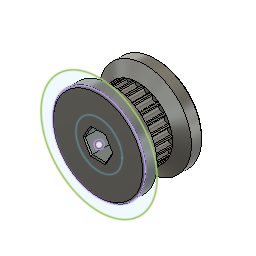
HTD Flanged Pulley (Autodesk Fusion 360 design; units mm, degrees)
Autodesk Fusion 360 part; units mm, degrees
sketch "Basic Outline" plane through (0, 0, 0) normal (0, 0, 1) x (1, 0, 0) in component "HTD 5M Pulley"
  circle A0 centre (0, 0) radius 18.5271
  line L0 (0, 0) -> (0, 17.9921) construction
  arc A1 (-1.525, 17.9914) -> (-2.0015, 18.4187) centre (-1.955, 17.9912) ccw
  arc A2 (-1.525, 17.9914) -> (1.525, 17.9914) centre (0, 17.9921) ccw
  arc A3 (2.0015, 18.4187) -> (1.525, 17.9914) centre (1.955, 17.9912) ccw
  dimension "d12" = 3.05
  dimension "d19" = 37.0542
  dimension "d20" = 16.4671
  dimension "d21" = 0.43
  constraint coincident A0.centre L0.start
  constraint coincident L0.end A2.centre
  constraint tangent A1 A2
  constraint tangent A0 A1
  constraint coincident A0 A1.end
  constraint vertical L0
  constraint tangent A0 A3
  constraint tangent A2 A3
  constraint coincident A0 A3.start
  constraint equal A1 A3
  measures "d12" diameter of A2
  measures "d19" diameter of A0
  measures "d20" distance of A0.centre A2
  measures "d21" radius of A1
extrude "Extrude1" add sketch "Basic Outline" along normal blind 5.5 in component "HTD 5M Pulley"
extrude "Extrude2" cut sketch "Basic Outline" along normal blind 5.5 contours A0 A1 A2 A3 picked at (-0.038, 17.8338) in component "HTD 5M Pulley"
pattern_circular "C-Pattern1" count 24 over 360 about axis through (0, 0, 1.75) along (0, 0, 1) of "Extrude2" in component "HTD 5M Pulley"
sketch "Flange" plane through (0, 0, 5.5) normal (0, 0, 1) x (1, 0, 0) in component "HTD 5M Pulley"
  arc A0 (2.0015, 18.4187) -> (1.525, 17.9914) centre (1.955, 17.9912) ccw
  arc A1 (-1.525, 17.9914) -> (1.525, 17.9914) centre (0, 17.9921) ccw
  arc A2 (-1.525, 17.9914) -> (-2.0015, 18.4187) centre (-1.955, 17.9912) ccw
  arc A3 (-2.0015, 18.4187) -> (-2.8338, 18.3091) centre (0, 0) ccw
  arc A4 (-2.8338, 18.3091) -> (-3.1835, 17.773) centre (-2.7681, 17.8841) ccw
  arc A5 (-6.1295, 16.9836) -> (-3.1835, 17.773) centre (-4.6567, 17.379) ccw
  arc A6 (-6.1295, 16.9836) -> (-6.7004, 17.2731) centre (-6.5448, 16.8722) ccw
  arc A7 (-6.7004, 17.2731) -> (-7.476, 16.9518) centre (0, 0) ccw
  arc A8 (-7.476, 16.9518) -> (-7.675, 16.3435) centre (-7.3025, 16.5583) ccw
  arc A9 (-10.3164, 14.8185) -> (-7.675, 16.3435) centre (-8.996, 15.5816) ccw
  arc A10 (-10.3164, 14.8185) -> (-10.9426, 14.9503) centre (-10.6887, 14.6033) ccw
  arc A11 (-10.9426, 14.9503) -> (-11.6087, 14.4392) centre (0, 0) ccw
  arc A12 (-11.6087, 14.4392) -> (-11.6435, 13.8002) centre (-11.3393, 14.1041) ccw
  arc A13 (-13.8002, 11.6435) -> (-11.6435, 13.8002) centre (-12.7223, 12.7223) ccw
  arc A14 (-13.8002, 11.6435) -> (-14.4392, 11.6087) centre (-14.1041, 11.3393) ccw
  arc A15 (-14.4392, 11.6087) -> (-14.9503, 10.9426) centre (0, 0) ccw
  arc A16 (-14.9503, 10.9426) -> (-14.8185, 10.3164) centre (-14.6033, 10.6887) ccw
  arc A17 (-16.3435, 7.675) -> (-14.8185, 10.3164) centre (-15.5816, 8.996) ccw
  arc A18 (-16.3435, 7.675) -> (-16.9518, 7.476) centre (-16.5583, 7.3025) ccw
  arc A19 (-16.9518, 7.476) -> (-17.2731, 6.7004) centre (0, 0) ccw
  arc A20 (-17.2731, 6.7004) -> (-16.9836, 6.1295) centre (-16.8722, 6.5448) ccw
  arc A21 (-17.773, 3.1835) -> (-16.9836, 6.1295) centre (-17.379, 4.6567) ccw
  arc A22 (-17.773, 3.1835) -> (-18.3091, 2.8338) centre (-17.8841, 2.7681) ccw
  arc A23 (-18.3091, 2.8338) -> (-18.4187, 2.0015) centre (0, 0) ccw
  arc A24 (-18.4187, 2.0015) -> (-17.9914, 1.525) centre (-17.9912, 1.955) ccw
  arc A25 (-17.9914, -1.525) -> (-17.9914, 1.525) centre (-17.9921, 0) ccw
  arc A26 (-17.9914, -1.525) -> (-18.4187, -2.0015) centre (-17.9912, -1.955) ccw
  arc A27 (-18.4187, -2.0015) -> (-18.3091, -2.8338) centre (0, 0) ccw
  arc A28 (-18.3091, -2.8338) -> (-17.773, -3.1835) centre (-17.8841, -2.7681) ccw
  arc A29 (-16.9836, -6.1295) -> (-17.773, -3.1835) centre (-17.379, -4.6567) ccw
  arc A30 (-16.9836, -6.1295) -> (-17.2731, -6.7004) centre (-16.8722, -6.5448) ccw
  arc A31 (-17.2731, -6.7004) -> (-16.9518, -7.476) centre (0, 0) ccw
  arc A32 (-16.9518, -7.476) -> (-16.3435, -7.675) centre (-16.5583, -7.3025) ccw
  arc A33 (-14.8185, -10.3164) -> (-16.3435, -7.675) centre (-15.5816, -8.996) ccw
  arc A34 (-14.8185, -10.3164) -> (-14.9503, -10.9426) centre (-14.6033, -10.6887) ccw
  arc A35 (-14.9503, -10.9426) -> (-14.4392, -11.6087) centre (0, 0) ccw
  arc A36 (-14.4392, -11.6087) -> (-13.8002, -11.6435) centre (-14.1041, -11.3393) ccw
  arc A37 (-11.6435, -13.8002) -> (-13.8002, -11.6435) centre (-12.7223, -12.7223) ccw
  arc A38 (-11.6435, -13.8002) -> (-11.6087, -14.4392) centre (-11.3393, -14.1041) ccw
  arc A39 (-11.6087, -14.4392) -> (-10.9426, -14.9503) centre (0, 0) ccw
  arc A40 (-10.9426, -14.9503) -> (-10.3164, -14.8185) centre (-10.6887, -14.6033) ccw
  arc A41 (-7.675, -16.3435) -> (-10.3164, -14.8185) centre (-8.996, -15.5816) ccw
  arc A42 (-7.675, -16.3435) -> (-7.476, -16.9518) centre (-7.3025, -16.5583) ccw
  arc A43 (-7.476, -16.9518) -> (-6.7004, -17.2731) centre (0, 0) ccw
  arc A44 (-6.7004, -17.2731) -> (-6.1295, -16.9836) centre (-6.5448, -16.8722) ccw
  arc A45 (-3.1835, -17.773) -> (-6.1295, -16.9836) centre (-4.6567, -17.379) ccw
  arc A46 (-3.1835, -17.773) -> (-2.8338, -18.3091) centre (-2.7681, -17.8841) ccw
  arc A47 (-2.8338, -18.3091) -> (-2.0015, -18.4187) centre (0, 0) ccw
  arc A48 (-2.0015, -18.4187) -> (-1.525, -17.9914) centre (-1.955, -17.9912) ccw
  arc A49 (1.525, -17.9914) -> (-1.525, -17.9914) centre (0, -17.9921) ccw
  arc A50 (1.525, -17.9914) -> (2.0015, -18.4187) centre (1.955, -17.9912) ccw
  arc A51 (2.0015, -18.4187) -> (2.8338, -18.3091) centre (0, 0) ccw
  arc A52 (2.8338, -18.3091) -> (3.1835, -17.773) centre (2.7681, -17.8841) ccw
  arc A53 (6.1295, -16.9836) -> (3.1835, -17.773) centre (4.6567, -17.379) ccw
  arc A54 (6.1295, -16.9836) -> (6.7004, -17.2731) centre (6.5448, -16.8722) ccw
  arc A55 (6.7004, -17.2731) -> (7.476, -16.9518) centre (0, 0) ccw
  arc A56 (7.476, -16.9518) -> (7.675, -16.3435) centre (7.3025, -16.5583) ccw
  arc A57 (10.3164, -14.8185) -> (7.675, -16.3435) centre (8.996, -15.5816) ccw
  arc A58 (10.3164, -14.8185) -> (10.9426, -14.9503) centre (10.6887, -14.6033) ccw
  arc A59 (10.9426, -14.9503) -> (11.6087, -14.4392) centre (0, 0) ccw
  arc A60 (11.6087, -14.4392) -> (11.6435, -13.8002) centre (11.3393, -14.1041) ccw
  arc A61 (13.8002, -11.6435) -> (11.6435, -13.8002) centre (12.7223, -12.7223) ccw
  arc A62 (13.8002, -11.6435) -> (14.4392, -11.6087) centre (14.1041, -11.3393) ccw
  arc A63 (14.4392, -11.6087) -> (14.9503, -10.9426) centre (0, 0) ccw
  arc A64 (14.9503, -10.9426) -> (14.8185, -10.3164) centre (14.6033, -10.6887) ccw
  arc A65 (16.3435, -7.675) -> (14.8185, -10.3164) centre (15.5816, -8.996) ccw
  arc A66 (16.3435, -7.675) -> (16.9518, -7.476) centre (16.5583, -7.3025) ccw
  arc A67 (16.9518, -7.476) -> (17.2731, -6.7004) centre (0, 0) ccw
  arc A68 (17.2731, -6.7004) -> (16.9836, -6.1295) centre (16.8722, -6.5448) ccw
  arc A69 (17.773, -3.1835) -> (16.9836, -6.1295) centre (17.379, -4.6567) ccw
  arc A70 (17.773, -3.1835) -> (18.3091, -2.8338) centre (17.8841, -2.7681) ccw
  arc A71 (18.3091, -2.8338) -> (18.4187, -2.0015) centre (0, 0) ccw
  arc A72 (18.4187, -2.0015) -> (17.9914, -1.525) centre (17.9912, -1.955) ccw
  arc A73 (17.9914, 1.525) -> (17.9914, -1.525) centre (17.9921, 0) ccw
  arc A74 (17.9914, 1.525) -> (18.4187, 2.0015) centre (17.9912, 1.955) ccw
  arc A75 (18.4187, 2.0015) -> (18.3091, 2.8338) centre (0, 0) ccw
  arc A76 (18.3091, 2.8338) -> (17.773, 3.1835) centre (17.8841, 2.7681) ccw
  arc A77 (16.9836, 6.1295) -> (17.773, 3.1835) centre (17.379, 4.6567) ccw
  arc A78 (16.9836, 6.1295) -> (17.2731, 6.7004) centre (16.8722, 6.5448) ccw
  arc A79 (17.2731, 6.7004) -> (16.9518, 7.476) centre (0, 0) ccw
  arc A80 (16.9518, 7.476) -> (16.3435, 7.675) centre (16.5583, 7.3025) ccw
  arc A81 (14.8185, 10.3164) -> (16.3435, 7.675) centre (15.5816, 8.996) ccw
  arc A82 (14.8185, 10.3164) -> (14.9503, 10.9426) centre (14.6033, 10.6887) ccw
  arc A83 (14.9503, 10.9426) -> (14.4392, 11.6087) centre (0, 0) ccw
  arc A84 (14.4392, 11.6087) -> (13.8002, 11.6435) centre (14.1041, 11.3393) ccw
  arc A85 (11.6435, 13.8002) -> (13.8002, 11.6435) centre (12.7223, 12.7223) ccw
  arc A86 (11.6435, 13.8002) -> (11.6087, 14.4392) centre (11.3393, 14.1041) ccw
  arc A87 (11.6087, 14.4392) -> (10.9426, 14.9503) centre (0, 0) ccw
  arc A88 (10.9426, 14.9503) -> (10.3164, 14.8185) centre (10.6887, 14.6033) ccw
  arc A89 (7.675, 16.3435) -> (10.3164, 14.8185) centre (8.996, 15.5816) ccw
  arc A90 (7.675, 16.3435) -> (7.476, 16.9518) centre (7.3025, 16.5583) ccw
  arc A91 (7.476, 16.9518) -> (6.7004, 17.2731) centre (0, 0) ccw
  arc A92 (6.7004, 17.2731) -> (6.1295, 16.9836) centre (6.5448, 16.8722) ccw
  arc A93 (3.1835, 17.773) -> (6.1295, 16.9836) centre (4.6567, 17.379) ccw
  arc A94 (3.1835, 17.773) -> (2.8338, 18.3091) centre (2.7681, 17.8841) ccw
  arc A95 (2.8338, 18.3091) -> (2.0015, 18.4187) centre (0, 0) ccw
  circle A96 centre (0, 0) radius 18.5271 construction
  circle A97 centre (0, 0) radius 25.0271
  circle A98 centre (0, 0) radius 75.0271
  dimension "d58" = 6.5
  dimension "d59" = 50
  constraint concentric A96 A97
  measures "d58" distance of A96 A97
  measures "d59" distance of A97 A98
extrude "Extrude3" add sketch "Basic Outline" along normal blind 10.15 draft 60 from surface at 5.5 in component "HTD 5M Pulley"
extrude "Extrude4" cut sketch "Flange" along normal through all contours A98 in component "HTD 5M Pulley"
sketch "Hub" plane through (0, 0, 15.65) normal (0, 0, 1) x (1, 0, 0) in component "HTD 5M Pulley"
  circle A0 centre (0, 0) radius 12.5
  circle A1 centre (0, 0) radius 31.3722
  circle A2 centre (0, 0) radius 25.0271
  dimension "d64" = 25
  measures "d64" diameter of A0
extrude "Extrude7" add sketch "Hub" along normal blind 0.6 contours A0 in component "HTD 5M Pulley"
sketch "Axle and Bolts" plane through (0, 0, 16.25) normal (0, 0, 1) x (1, 0, 0) in component "HTD 5M Pulley"
  circle A0 centre (0, 0) radius 18.5271 construction
  line L0 (-3.7212, 6.4452) -> (-7.4423, 0)
  line L1 (-7.4423, 0) -> (-3.7212, -6.4453)
  line L2 (-3.7212, -6.4453) -> (3.7212, -6.4453)
  line L3 (3.7212, -6.4452) -> (7.4423, 0)
  line L4 (7.4423, 0) -> (3.7212, 6.4452)
  line L5 (3.7212, 6.4452) -> (-3.7212, 6.4452)
  circle A1 centre (0, 0) radius 21.0271
  line L6 (0, 0) -> (0, 11.9671) construction
  circle A2 centre (0, 0) radius 15
  circle A3 centre (0, 0) radius 12.5
  line L7 (3.7212, -6.4452) -> (7.5, -12.9904) construction
  line L8 (5.6106, -9.7178) -> (11.2212, 0)
  line L9 (11.2212, 0) -> (5.6106, 9.7178)
  line L10 (5.6106, 9.7178) -> (-5.6106, 9.7178)
  line L11 (-5.6106, 9.7178) -> (-11.2212, 0)
  line L12 (-11.2212, 0) -> (-5.6106, -9.7178)
  line L13 (-5.6106, -9.7178) -> (5.6106, -9.7178)
  line L14 (12.6068, 0) -> (6.3034, 10.9178)
  line L15 (6.3034, 10.9178) -> (-6.3034, 10.9178)
  line L16 (-6.3034, 10.9178) -> (-12.6068, 0)
  line L17 (-12.6068, 0) -> (-6.3034, -10.9178)
  line L18 (-6.3034, -10.9178) -> (6.3034, -10.9178)
  line L19 (6.3034, -10.9178) -> (12.6068, 0)
  point P0 (0, 11.9671)
  dimension "d60" = 6.4452
  dimension "d77" = 11.9671
  dimension "d83" = 1.2
  constraint coincident A0.centre A1.centre
  constraint coincident P0 L6.end
  constraint perpendicular L5 L6
  constraint vertical L6
  constraint coincident A2 L7.end
  constraint parallel L1 L7
  constraint coincident L7 L8.start
  constraint midpoint L7 L8.start
  measures "d60" distance of A0.centre L5
  measures "d77" distance of A0.centre L6.end
extrude "Extrude6" cut sketch "Axle and Bolts" against normal through all contours L0 L1 L2 L3 L4 L5 in component "HTD 5M Pulley"
chamfer "Chamfer1" distance 0.6 angle 45 6 edges at (5.5818, -3.2226, 16.25) (0, -6.4453, 16.25) (-5.5818, -3.2226, 16.25) (-5.5818, 3.2226, 16.25) (0, 6.4452, 16.25) (5.5818, 3.2226, 16.25) in component "HTD 5M Pulley"
mirror "Mirror1" about plane through (0, 0, 0) normal (0, 0, -1) of bodies 1 merged in component "HTD 5M Pulley"
extrude "Extrude9" add sketch "Hub" along normal up to surface (0.6 mm away) contours A2 in component "HTD 5M Pulley"
chamfer "Chamfer2" distance 0.9 angle 45 2 edges at (-23.3334, 9.0502, 16.25) (-23.3334, -9.0502, -15.65) in component "HTD 5M Pulley"
component "HTD 5M Pulley" placed x (1, 0, 0) y (0, 1, 0) z (0, 0, 1) at (0, 0, 0)
equation "NUM_TEETH = 24" comment "Number of teeth in the pulley"
equation "TOOTH_PITCH = 5 mm" comment "Belt pitch (ie: 5mm=HTD5)"
equation "zOutsideDia = 2 * ( ( NUM_TEETH * TOOTH_PITCH ) / ( PI * 2 ) - zPitchLineOffset )"
equation "zPitchLineOffset = 0.5715 mm"
equation "zToothDia = 2.06 mm"
equation "zMinorDia = zOutsideDia - 2 * zToothDia"
equation "zToothWidth = 3.05 mm"
equation "zToothRootDia = 0.86 mm"
equation "d12 = zToothWidth"
equation "d17 = TOOTH_WIDTH / 2"
equation "d19 = zOutsideDia"
equation "d20 = zMinorDia / 2"
equation "d21 = zToothRootDia / 2"
equation "d22 = d17"
equation "d24 = NUM_TEETH"
equation "TOOTH_WIDTH = 11 mm" comment "Width of the toothed part of the pulley"
equation "TOTAL_WIDTH = 14.5 mm + EXTRA_WIDTH" comment "Total width of the pulley at the hub"
equation "PRINTER_LAYER_HEIGHT = 0.3 mm" comment "Layer height of printer (typically 0.2mm or 0.3mm)"
equation "HUB_OFFSET = if(PRINTER_LAYER_HEIGHT >= 0.3 mm; PRINTER_LAYER_HEIGHT * 2; PRINTER_LAYER_HEIGHT * 3)" comment "Distant hub projects above rim (so rim won't scrape when pulley rotates)"
equation "FLANGE_ANGLE = 60 deg" comment "Typically 60 if printing with a hub offset, 80 otherwise"
equation "HEX_SHAFT_DIAMETER = 0.5075 in" comment "Hex shaft diameter + tolerance"
equation "d34 = ( TOTAL_WIDTH - TOOTH_WIDTH ) / 2 - HUB_OFFSET"
equation "d35 = FLANGE_ANGLE"
equation "FLANGE_MAX_HEIGHT = 2.5 mm + EXTRA_DIAMETER" comment "Max height of the flange"
equation "HUB_DIAMETER = 25 mm" comment "Diameter of the raised hub"
equation "NUM_BOLTS = 6" comment "Number of mounting bolts (edit feature to change type)"
equation "d54 = PRINTER_LAYER_HEIGHT * 2"
equation "d58 = FLANGE_MAX_HEIGHT"
equation "d60 = HEX_SHAFT_DIAMETER / 2"
equation "BOLT_RADIUS = min(( zOutsideDia + HUB_DIAMETER ) / 4; zMinorDia / 2 - 4.5 mm)" comment "Radius of the bolt circle (default is halfway between hub and rim)"
equation "d64 = HUB_DIAMETER"
equation "d65 = HUB_OFFSET"
equation "d77 = BOLT_RADIUS"
equation "PRINTER_NOZZLE_DIAMETER = 0.6 mm" comment "Nozzle Diameter"
equation "PRINTER_TOLERANCE_MED = 0.005 in" comment "Offset for groove"
equation "d83 = PRINTER_NOZZLE_DIAMETER * 2"
equation "EXTRA_WIDTH = 18 mm" comment "Extra flange width"
equation "EXTRA_DIAMETER = 4 mm" comment "Extra diameter for robustness (over standard)"
equation "d94 = PRINTER_LAYER_HEIGHT * 3"
named bodies: "Male"
